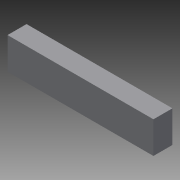
# Autodesk Inventor part: BumperFront
Saved by Autodesk Inventor 2013 (Build 170138000, 138)
## iProperties
Created: 2014-01-09
Part Number: BumperFront
Material: Generic
Document SubType Name: Modeling
Designer: 215152
Density: 1 g/cm^3
Author: 215152
Autodesk Inventor part; units mm, degrees
ref_plane "YZ Plane" through (0, 0, 0) normal (1, 0, 0) x (0, 1, 0)
ref_plane "XZ Plane" through (0, 0, 0) normal (0, 1, 0) x (-1, 0, 0)
ref_plane "XY Plane" through (0, 0, 0) normal (0, 0, 1) x (1, 0, 0)
sketch "Sketch1" plane through (0, 0, 0) normal (0, 0, 1) x (1, 0, 0)
  line L0 (0, 0) -> (-92.075, 0)
  line L1 (-92.075, 0) -> (-92.075, 25.4)
  line L2 (-92.075, 25.4) -> (-92.075, -101.6)
  line L3 (-92.075, -101.6) -> (492.125, -101.6)
  line L4 (492.125, -101.6) -> (492.125, 25.4)
  line L5 (492.125, 25.4) -> (-92.075, 25.4)
  dimension "d0" = 92.075
  dimension "d1" = 25.4
  dimension "d2" = 127
  dimension "d3" = 0
  dimension "d4" = 584.2
  dimension "d5" = 90
  dimension "d6" = 127
  dimension "d7" = 90
  constraints: 12 end point, 2 parallel, 1 collinear, 1 horizontal, 1 perpendicular
  measures "d0" distance of L0.start L0.end
  measures "d1" distance of L0.end L1.end
  measures "d2" distance of L1.end L2.end
  measures "d3" distance between parallel lines of L2 L1
  measures "d4" distance of L2.end L3.end
  measures "d5" angle of L3 L2
  measures "d6" distance of L3.end L4.end
  measures "d7" angle of L4 L3
extrude "Extrusion1" add sketch "Sketch1" along normal blind 76.2
body "Solid1"
